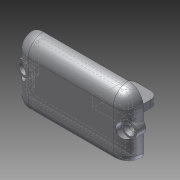
# Autodesk Inventor part: x-IMU 2 Housing - Main
Saved by Autodesk Inventor 2012 (Build 160160000, 160)
## iProperties
Created: 2011-08-17
Part Number: x-IMU 2 Housing - Main
Document SubType Name: Modeling
Designer: Jacky
Density: 1 g/cm^3
Material: Default
Author: Jacky
Autodesk Inventor part; units mm, degrees
ref_plane "YZ Plane" through (0, 0, 0) normal (1, 0, 0) x (0, 1, 0)
sketch "Sketch1" plane through (0, 0, 0) normal (0, 0, 1) x (1, 0, 0)
  line L0 (-19, 10.3) -> (19, 10.3)
  line L1 (19, 10.3) -> (19, -10.3)
  line L2 (19, -10.3) -> (-19, -10.3)
  line L3 (-19, -10.3) -> (-19, 10.3)
  point P0 (0, 0)
  point P1 (19, 0)
  point P2 (0, 10.3)
  dimension "d0" = 38
  dimension "d1" = 20.6
  constraints: 8 end point, 2 midpoint, 2 parallel, 1 horizontal, 1 horizontal alignment, 1 perpendicular, 1 vertical alignment
  measures "d0" distance between parallel lines of L1 L3
  measures "d1" distance of L0.end L1.end
extrude "Extrusion_Main" add sketch "Sketch1" along normal blind 28.5 and the other way blind 28.5
fillet "Fillet_Main" radius 5 8 edges at (19, 10.3, 0) (19, 0, 28.5) (0, 10.3, 28.5) (-19, 0, 28.5) (-19, 10.3, 0) (19, 0, -28.5) (0, 10.3, -28.5) (-19, 0, -28.5)
fillet "Fillet_Main_bottom" radius 2.5 8 edges at (0, -10.3, 28.5) (-17.5355, -10.3, 27.0355) (-19, -10.3, 0) (-17.5355, -10.3, -27.0355) (0, -10.3, -28.5) (17.5355, -10.3, -27.0355) (19, -10.3, 0) (17.5355, -10.3, 27.0355)
ref_plane "Work Plane2" through (0, 0, 26.5) normal (0, 0, 1) x (1, 0, 0)
sketch "Sketch7" plane through (0, 0, 26.5) normal (0, 0, 1) x (1, 0, 0)
  line L0 (19, -7.8) -> (14, -7.8) projected
  line L1 (19, -7.8) -> (19, 5.3) projected
  line L2 (19, 5.3) -> (14, 5.3) projected
  line L3 (14, 5.3) -> (14, -7.8) projected
  line L4 (19, 5.3) -> (14, 5.3) projected
  arc A0 (19, 5.3) -> (14, 10.3) centre (14, 5.3) ccw projected
  line L5 (14, 5.3) -> (14, 10.3) projected
  line L6 (14, 5.3) -> (14, 10.3) projected
  line L7 (14, 10.3) -> (-14, 10.3) projected
  line L8 (-14, 10.3) -> (-14, 5.3) projected
  line L9 (-14, 5.3) -> (14, 5.3) projected
  line L10 (14, -7.8) -> (14, -10.3) projected
  line L11 (14, -10.3) -> (-14, -10.3) projected
  line L12 (-14, -7.8) -> (-14, -10.3) projected
  line L13 (-14, -7.8) -> (14, -7.8) projected
  arc A1 (16.5, -10.3) -> (19, -7.8) centre (16.5, -7.8) ccw projected
  line L14 (16.5, -10.3) -> (14, -10.3) projected
  line L15 (14, -7.8) -> (14, -10.3) projected
  line L16 (14, -7.8) -> (19, -7.8) projected
  circle A2 centre (17.25, -0.375) radius 2.5
  point P0 (0, 0)
  dimension "d33" = 5
  dimension "d34" = 9.925
  dimension "d35" = 1.75
  constraints: 1 centre point
  measures "d33" diameter of A2
  measures "d34" distance from line of L11 A2.centre
  measures "d35" distance from line of L1 A2.centre
extrude "Extrusion_screwHeadSupport" add sketch "Sketch7" against normal blind 8 contours A2 L1 | L1 A2
fillet "Fillet_screwHeadSupport" radius 2 1 edges at (19.75, -0.375, 18.5)
sketch "Sketch8" plane through (0, 0, 26.5) normal (0, 0, 1) x (1, 0, 0)
  arc A0 (18, -2.7598) -> (18, 2.0098) centre (17.25, -0.375) ccw projected
  circle A1 centre (17.25, -0.375) radius 2.5
  point P0 (0, 0)
  constraints: 1 centre point, 1 coincident, 1 concentric
extrude "Extrusion_screwHeadSupport_clearance" cut sketch "Sketch8" along normal blind 8
sketch "Sketch9" plane through (0, 0, 26.5) normal (0, 0, 1) x (1, 0, 0)
  arc A0 (18, -2.7598) -> (18, 2.0098) centre (17.25, -0.375) ccw projected
  point P0 (0, 0)
hole "Hole_screw" at (17.25, -0.375, 26.5) direction (0, 0, -1) diameter 1.8 depth 6 tip angle 120 countersink diameter 3.8 countersink angle 90
sketch "Sketch10" plane through (0, 0, 26.5) normal (0, 0, 1) x (1, 0, 0)
  arc A0 (18, 2.0098) -> (18, -2.7598) centre (17.25, -0.375) ccw projected
  circle A1 centre (17.25, -0.375) radius 1
  point P0 (0, 0)
  dimension "d47" = 2
  constraints: 1 centre point, 1 coincident
  measures "d47" diameter of A1
extrude "Extrusion_screwClearance" cut sketch "Sketch10" against normal blind 3
mirror "Mirror_screwLeftRight" about plane through (0, 0, 0) normal (1, 0, 0) of "Extrusion_screwHeadSupport", "Fillet_screwHeadSupport", "Extrusion_screwHeadSupport_clearance", "Hole_screw", "Extrusion_screwClearance"
sketch "Sketch11" plane through (-14, 10.3, -23.5) normal (0, 1, 0) x (1, 0, 0)
  line L0 (28, 0) -> (28, -47) projected
  line L1 (0, 0) -> (28, 0) projected
  line L2 (0, -47) -> (0, 0) projected
  line L3 (28, -47) -> (0, -47) projected
  circle A0 centre (6, -24) radius 1
  circle A1 centre (6, -24) radius 2
  circle A2 centre (6, -24) radius 3
  arc A3 (6.5, -29) -> (5.5, -29) centre (6, -29) ccw
  line L4 (5.5, -29) -> (5.5, -41)
  line L5 (5.5, -41) -> (4.309, -39.299)
  arc A4 (4.309, -39.299) -> (3.4898, -39.8726) centre (3.8994, -39.5858) ccw
  arc A5 (5.5904, -42.8726) -> (6.4096, -42.8726) centre (6, -42.5858) ccw
  line L6 (3.4898, -39.8726) -> (5.5904, -42.8726)
  line L7 (6.5, -29) -> (6.5, -41)
  line L8 (6.5, -41) -> (7.8546, -39.0654)
  arc A6 (8.564, -39.7957) -> (7.8546, -39.0654) centre (8.2093, -39.4306) ccw
  line L9 (8.564, -39.7957) -> (6.4096, -42.8726)
  arc A7 (11, -23.5) -> (11, -24.5) centre (11, -24) ccw
  line L10 (11, -24.5) -> (23, -24.5)
  line L11 (23, -24.5) -> (21.299, -25.691)
  arc A8 (21.299, -25.691) -> (21.8726, -26.5102) centre (21.5858, -26.1006) ccw
  arc A9 (24.8726, -24.4096) -> (24.8726, -23.5904) centre (24.5858, -24) ccw
  line L12 (21.8726, -26.5102) -> (24.8726, -24.4096)
  line L13 (21.7957, -21.436) -> (24.8726, -23.5904)
  line L14 (23, -23.5) -> (21.0654, -22.1454)
  arc A10 (21.7957, -21.436) -> (21.0654, -22.1454) centre (21.4306, -21.7907) ccw
  line L15 (11, -23.5) -> (23, -23.5)
  line L16 (24.5858, -32) -> (21.5858, -32) construction
  line L17 (21.5858, -32) -> (21.5858, -29) construction
  line L18 (21.5858, -29) -> (24.5858, -29) construction
  line L19 (24.5858, -29) -> (24.5858, -32) construction
  line L20 (11, -39.4306) -> (14, -39.4306) construction
  line L21 (14, -39.4306) -> (14, -42.4306) construction
  line L22 (14, -42.4306) -> (11, -42.4306) construction
  line L23 (11, -42.4306) -> (11, -39.4306) construction
  line L24 (11, -29) -> (14, -29) construction
  line L25 (14, -29) -> (14, -32) construction
  line L26 (14, -32) -> (11, -32) construction
  line L27 (11, -32) -> (11, -29) construction
  line L28 (19, -6) -> (16, -6) construction
  line L29 (16, -6) -> (16, -3) construction
  line L30 (16, -3) -> (19, -3) construction
  line L31 (19, -3) -> (19, -6) construction
  line L32 (13.904, -32.25) -> (11.1301, -32.25)
  line L33 (11.1301, -32.25) -> (11.1301, -31.5948)
  line L34 (11.1301, -31.5948) -> (12.7439, -29.4165)
  line L35 (12.7439, -29.4165) -> (11.2152, -29.4165)
  line L36 (11.2152, -29.4165) -> (11.2152, -28.75)
  line L37 (11.2152, -28.75) -> (13.8104, -28.75)
  line L38 (13.8104, -28.75) -> (13.8104, -29.4165)
  line L39 (13.8104, -29.4165) -> (12.2022, -31.5835)
  line L40 (12.2022, -31.5835) -> (13.904, -31.5835)
  line L41 (13.904, -31.5835) -> (13.904, -32.25)
  line L42 (14.1479, -42.6806) -> (13.1325, -42.6806)
  line L43 (13.1325, -42.6806) -> (12.4575, -41.5659)
  line L44 (12.4575, -41.5659) -> (11.7682, -42.6806)
  line L45 (11.7682, -42.6806) -> (10.7954, -42.6806)
  line L46 (10.7954, -42.6806) -> (11.9327, -40.9192)
  line L47 (11.9327, -40.9192) -> (10.8408, -39.1806)
  line L48 (10.8408, -39.1806) -> (11.8562, -39.1806)
  line L49 (11.8562, -39.1806) -> (12.4887, -40.2385)
  line L50 (12.4887, -40.2385) -> (13.1382, -39.1806)
  line L51 (13.1382, -39.1806) -> (14.111, -39.1806)
  line L52 (14.111, -39.1806) -> (13.0134, -40.8823)
  line L53 (13.0134, -40.8823) -> (14.1479, -42.6806)
  line L54 (21.4705, -32.25) -> (22.6788, -30.2107)
  line L55 (22.6788, -30.2107) -> (22.6788, -28.75)
  line L56 (22.6788, -28.75) -> (23.558, -28.75)
  line L57 (23.558, -28.75) -> (23.558, -30.1682)
  line L58 (23.558, -30.1682) -> (24.7862, -32.25)
  line L59 (24.7862, -32.25) -> (23.7849, -32.25)
  line L60 (23.7849, -32.25) -> (23.1014, -31.002)
  line L61 (23.1014, -31.002) -> (22.4405, -32.25)
  line L62 (22.4405, -32.25) -> (21.4705, -32.25)
  line L63 (22.1657, -2.7869) -> (23.1301, -2.7869)
  line L64 (23.1301, -2.7869) -> (23.6321, -3.5442)
  line L65 (23.6321, -3.5442) -> (24.1483, -2.7869)
  line L66 (24.1483, -2.7869) -> (25.0928, -2.7869)
  line L67 (25.0928, -2.7869) -> (24.1199, -4.1086)
  line L68 (24.1199, -4.1086) -> (25.0758, -5.4275)
  line L69 (25.0758, -5.4275) -> (24.1114, -5.4275)
  line L70 (24.1114, -5.4275) -> (23.6179, -4.6844)
  line L71 (23.6179, -4.6844) -> (23.1216, -5.4275)
  line L72 (23.1216, -5.4275) -> (22.1771, -5.4275)
  line L73 (22.1771, -5.4275) -> (23.1329, -4.1284)
  line L74 (23.1329, -4.1284) -> (22.1657, -2.7869)
  line L75 (20.359, -4.0065) -> (21.9161, -4.0065)
  line L76 (21.9161, -4.0065) -> (21.9161, -4.6588)
  line L77 (21.9161, -4.6588) -> (20.359, -4.6588)
  line L78 (20.359, -4.6588) -> (20.359, -4.0065)
  line L79 (17.9935, -2.7869) -> (19.8768, -2.7869)
  line L80 (19.8768, -2.7869) -> (19.8768, -3.3967)
  line L81 (19.8768, -3.3967) -> (19.3748, -3.3967)
  line L82 (19.3748, -3.3967) -> (19.3748, -5.6771)
  line L83 (19.3748, -5.6771) -> (19.8768, -5.6771)
  line L84 (19.8768, -5.6771) -> (19.8768, -6.2869)
  line L85 (19.8768, -6.2869) -> (17.9935, -6.2869)
  line L86 (17.9935, -6.2869) -> (17.9935, -5.6771)
  line L87 (17.9935, -5.6771) -> (18.4955, -5.6771)
  line L88 (18.4955, -5.6771) -> (18.4955, -3.3967)
  line L89 (18.4955, -3.3967) -> (17.9935, -3.3967)
  line L90 (17.9935, -3.3967) -> (17.9935, -2.7869)
  line L91 (13.8355, -2.7869) -> (14.7091, -2.7869)
  line L92 (14.7091, -2.7869) -> (14.7091, -5.107)
  line L93 (14.7091, -5.107) -> (15.3444, -3.6094)
  line L94 (15.3444, -3.6094) -> (15.9457, -3.6094)
  line L95 (15.9457, -3.6094) -> (16.581, -5.107)
  line L96 (16.581, -5.107) -> (16.581, -2.7869)
  line L97 (16.581, -2.7869) -> (17.4092, -2.7869)
  line L98 (17.4092, -2.7869) -> (17.4092, -6.2869)
  line L99 (17.4092, -6.2869) -> (16.3967, -6.2869)
  line L100 (16.3967, -6.2869) -> (15.6195, -4.5596)
  line L101 (15.6195, -4.5596) -> (14.8481, -6.2869)
  line L102 (14.8481, -6.2869) -> (13.8355, -6.2869)
  line L103 (13.8355, -6.2869) -> (13.8355, -2.7869)
  spline S0 degree 2 poles (11.6941, -2.7131) (12.4003, -2.7131) (13.1605, -3.3938) (13.1605, -4.0519) knots 0 0 0 1 2 2 2
  line L104 (13.1605, -4.0519) -> (13.1605, -6.2869)
  line L105 (13.1605, -6.2869) -> (12.2812, -6.2869)
  line L106 (12.2812, -6.2869) -> (12.2812, -4.1029)
  spline S1 degree 2 poles (12.2812, -4.1029) (12.2812, -3.737) (12.0061, -3.3797) (11.6941, -3.3797) knots 0 0 0 1 2 2 2
  spline S2 degree 2 poles (11.6941, -3.3797) (11.3906, -3.3797) (11.107, -3.7229) (11.107, -4.1029) knots 0 0 0 1 2 2 2
  line L107 (11.107, -4.1029) -> (11.107, -6.2869)
  line L108 (11.107, -6.2869) -> (10.2277, -6.2869)
  line L109 (10.2277, -6.2869) -> (10.2277, -4.0547)
  spline S3 degree 2 poles (10.2277, -4.0547) (10.2277, -3.408) (10.968, -2.7131) (11.6941, -2.7131) knots 0 0 0 1 2 2 2
  point P0 (14, -23.5)
  dimension "d51" = 2
  dimension "d54" = 1
  dimension "d55" = 1
  dimension "d56" = 1
  dimension "d57" = 5
  dimension "d58" = 12
  dimension "d59" = 35
  dimension "d60" = 1
  dimension "d61" = 1
  dimension "d62" = 3
  dimension "d65" = 90
  dimension "d67" = 6
  dimension "d68" = 6
  dimension "d69" = 3
  dimension "d70" = 3
  dimension "d72" = 3
  dimension "d73" = 3
  dimension "d74" = 3
  dimension "d75" = 3
  dimension "d76" = 3
  dimension "d77" = 3
  dimension "d78" = 3
  dimension "d79" = 5
  dimension "d80" = 5
  dimension "d81" = 5
  dimension "d82" = 5
  dimension "d83" = 0
  dimension "d84" = 3
  dimension "d85" = 24
  dimension "d86" = 9
  constraints: 24 end point, 16 point on circle, 11 centre point, 4 tangent, 2 coincident, 1 parallel, 1 perpendicular, 1 vertical alignment, 33 other
  measures "d51" diameter of A0
  measures "d54" radial gap between concentric circles of A1 A0
  measures "d55" radial gap between concentric circles of A2 A1
  measures "d56" diameter of A3
  measures "d57" distance of A0.centre A3.centre
  measures "d58" distance of L4.start L4.end
  measures "d59" angle of L4 L5
  measures "d60" diameter of A4
  measures "d61" diameter of A5
  measures "d62" vertical distance of A4.centre A5.centre
  measures "d67" distance from line of L2 A3.centre
  measures "d68" distance from line of L2 A0.centre
  measures "d69" distance between parallel lines of L23 L21
  measures "d70" distance between parallel lines of L17 L19
  measures "d72" distance between parallel lines of L20 L22
  measures "d73" distance between parallel lines of L16 L18
  measures "d74" distance between parallel lines of L25 L27
  measures "d75" distance between parallel lines of L24 L26
  measures "d76" distance of L30.end L28.start
  measures "d77" distance between parallel lines of L31 L29
  measures "d78" distance from line of A6.centre L22
  measures "d79" distance from line of A5.centre L23
  measures "d80" distance from line of A3.centre L27
  measures "d81" distance from line of A7.centre L24
  measures "d82" distance from line of L18 A9.centre
  measures "d83" distance from line of A9.centre L19
  measures "d84" distance between parallel lines of L1 L30
  measures "d85" distance from line of L1 A9.centre
  measures "d86" distance between parallel lines of L0 L31
extrude "Extrusion_text" cut sketch "Sketch11" against normal blind 0.5 contours A0 | A2 | L7 L8 A6 L9 A5 L6 A4 L5 L4 A3 | L15 L14 A10 L13 A9 L12 A8 L11 L10 A7 | L32 L33 L34 L35 L36 L37 L38 L39 L40 L41 | L42 L43 L44 L45 L46 L47 L48 L49 L50 L51 L52 L53 | L54 L55 L56 L57 L58 L59 L60 L61 L62 | L63 L64 L65 L66 L67 L68 L69 L70 L71 L72 L73 L74 | L75 L76 L77 L78 | L79 L80 L81 L82 L83 L84 L85 L86 L87 L88 L89 L90 | L91 L92 L93 L94 L95 L96 L97 L98 L99 L100 L101 L102 L103 | S0 L104 L105 L106 S1 S2 L107 L108 L109 S3
ref_plane "Work Plane4" through (14, 10.3, 23.5) normal (0, 0, 1) x (-1, 0, 0)
sketch "Sketch15" plane through (14, 10.3, 23.5) normal (0, 0, 1) x (-1, 0, 0)
  line L0 (37.3275, -2.4965) -> (-12.3019, -2.4965)
  line L1 (-12.3019, -2.4965) -> (-12.3019, 24.1032)
  line L2 (-12.3019, 24.1032) -> (37.3275, 24.1032)
  line L3 (37.3275, 24.1032) -> (37.3275, -2.4965)
  point P0 (14, 10.3)
  constraints: 8 end point, 2 parallel, 1 horizontal, 1 perpendicular
extrude "Extrusion_Mainvoid" cut sketch "Sketch15" against normal through all
sketch "Sketch16" plane through (14, 10.3, 23.5) normal (0, 0, -1) x (-1, 0, 0)
  line L0 (-5, -8.8896) -> (-5, -5) projected
  line L1 (-5, -18.1) -> (-5, -12.4604) projected
  line L2 (30.5, -20.6) -> (-2.5, -20.6) projected
  line L3 (33, -12.4604) -> (33, -18.1) projected
  line L4 (33, -5) -> (33, -8.8896) projected
  line L5 (0, 0) -> (28, 0) projected
  line L6 (-3.5, -19.6) -> (31.5, -19.6)
  line L7 (31.5, -19.6) -> (31.5, -13.1)
  line L8 (-3.5, -19.6) -> (-3.5, -13.1)
  line L9 (-3.5, -13.1) -> (-1.5, -13.1)
  line L10 (-1.5, -13.1) -> (-1.5, -2)
  line L11 (-1.5, -2) -> (29.5, -2)
  line L12 (29.5, -2) -> (29.5, -13.1)
  line L13 (29.5, -13.1) -> (31.5, -13.1)
  point P0 (14, -10.3)
  dimension "d93" = 6.5
  dimension "d94" = 1.5
  dimension "d95" = 6.5
  dimension "d96" = 1.5
  dimension "d97" = 1
  dimension "d98" = 2
  dimension "d99" = 3.5
  dimension "d100" = 3.5
  constraints: 16 end point, 4 parallel, 3 perpendicular, 1 collinear
  measures "d93" distance of L6.end L7.end
  measures "d94" distance between parallel lines of L3 L7
  measures "d95" distance of L6.start L8.end
  measures "d96" distance between parallel lines of L1 L8
  measures "d97" distance between parallel lines of L2 L6
  measures "d98" distance between parallel lines of L5 L11
  measures "d99" distance between parallel lines of L0 L10
  measures "d100" distance between parallel lines of L4 L12
extrude "Extrusion_internal" cut sketch "Sketch16" against normal blind 2.82
sketch "Sketch17" plane through (14, 10.3, 26.32) normal (0, 0, -1) x (-1, 0, 0)
  line L0 (-3.5, -19.6) -> (31.5, -19.6) projected
  line L1 (-5, -8.8896) -> (-5, -5) projected
  line L2 (31.5, -13.1) -> (31.5, -19.6) projected
  line L3 (31.5, -19.6) -> (-3.5, -19.6) projected
  line L4 (-3.5, -19.6) -> (-3.5, -13.1) projected
  line L5 (-3.5, -13.1) -> (-1.5, -13.1) projected
  line L6 (-1.5, -13.1) -> (-1.5, -2) projected
  line L7 (-1.5, -2) -> (29.5, -2) projected
  line L8 (29.5, -2) -> (29.5, -13.1) projected
  line L9 (29.5, -13.1) -> (31.5, -13.1) projected
  circle A0 centre (31.25, -10.675) radius 1 projected
  circle A1 centre (-3.25, -10.675) radius 1 projected
  line L10 (-5, -8.8896) -> (-5, -5) projected
  arc A2 (-5, -8.8896) -> (-5, -12.4604) centre (-3.25, -10.675) ccw projected
  line L11 (-5, -18.1) -> (-5, -12.4604) projected
  arc A3 (-5, -18.1) -> (-2.5, -20.6) centre (-2.5, -18.1) ccw projected
  line L12 (30.5, -20.6) -> (-2.5, -20.6) projected
  arc A4 (30.5, -20.6) -> (33, -18.1) centre (30.5, -18.1) ccw projected
  line L13 (33, -12.4604) -> (33, -18.1) projected
  arc A5 (33, -12.4604) -> (33, -8.8896) centre (31.25, -10.675) ccw projected
  line L14 (33, -5) -> (33, -8.8896) projected
  arc A6 (33, -5) -> (28, 0) centre (28, -5) ccw projected
  line L15 (0, 0) -> (28, 0) projected
  arc A7 (0, 0) -> (-5, -5) centre (0, -5) ccw projected
  line L16 (-2.2, -6.85) -> (-2.2, -9.25)
  line L17 (-2.2, -6.85) -> (7.4, -6.85)
  line L18 (7.4, -6.85) -> (7.4, -9.25)
  line L19 (7.4, -9.25) -> (-2.2, -9.25)
  line L20 (-2.2, -9.25) -> (-2.2, -6.85)
  point P0 (14, -10.3)
  point P1 (-3.4825, -19.6)
  point P2 (31.4825, -19.6)
  dimension "d103" = 2.4
  dimension "d104" = 2.8
  dimension "d105" = 9.6
  dimension "d106" = 10.35
  dimension "d107" = 2.4
  constraints: 10 end point, 2 parallel, 2 perpendicular, 1 horizontal
  measures "d103" distance of L16.start L16.end
  measures "d104" distance between parallel lines of L16 L1
  measures "d105" distance of L18.end L19.end
  measures "d106" distance between parallel lines of L0 L19
  measures "d107" distance of L17.end L18.end
extrude "Extrusion_PCBstay" add sketch "Sketch17" along normal blind 10.57 contours L19 L16 L17 L6 | L6 L17 L18 L19
fillet "Fillet_PSBstay" radius 2.5 2 edges at (16.2, 2.25, 15.75) (6.6, 2.25, 15.75)
fillet "Fillet_internal" radius 1.5 19 edges at (0, 8.3, 26.32) (-15.5, 8.3, 24.91) (-15.5, 2.75, 26.32) (-16.5, -2.8, 26.32) (-17.5, -2.8, 24.91) (-17.5, -6.05, 26.32) (-17.5, -9.3, 24.91) (0, -9.3, 26.32) (17.5, -6.05, 26.32) (17.5, -9.3, 24.91) (17.5, -2.8, 24.91) (16.5, -2.8, 26.32) (15.5, -0.875, 26.32) (15.5, 8.3, 24.91) (15.5, 5.875, 26.32) (11.05, 1.05, 26.32) (6.6, 2.25, 26.32) (11.05, 3.45, 26.32) (15.5, 1.05, 24.91)
equation "\"d60\" = d56"
equation "\"d61\" = d60"
equation "\"d67\" = d68"
equation "\"d93\" = d95"
body "Solid1"
